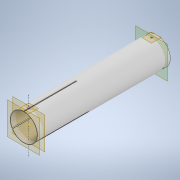
# Autodesk Inventor part: Segment_Engine
Saved by Autodesk Inventor 2020 (Build 240168000, 168)
## iProperties
Created: 2022-01-25
Part Number: Segment_Engine
Material: Generisch
Document SubType Name: Modeling
Designer: sp
Density: 1 g/cm^3
Appearance: Vorgabe
Author: sp
Autodesk Inventor part; units mm, degrees
ref_plane "YZ Plane" through (0, 0, 0) normal (1, 0, 0) x (0, 1, 0)
ref_plane "XZ Plane" through (0, 0, 0) normal (0, 1, 0) x (-1, 0, 0)
sketch "Skizze1" plane through (0, 0, 0) normal (0, 0, 1) x (1, 0, 0)
  circle A0 centre (0, 0) radius 31
  circle A1 centre (0, 0) radius 30
  dimension "d0" = 62
  dimension "d1" = 60
  constraints: 2 centre point, 2 coincident
  measures "d0" diameter of A0
  measures "d1" diameter of A1
extrude "Extrusion1" add sketch "Skizze1" along normal mid plane 300
ref_plane "Arbeitsebene1" through (0, 0, 138.75) normal (0, 0, 1) x (1, 0, 0)
sketch "Skizze2" plane through (0, 0, 138.75) normal (0, 0, 1) x (1, 0, 0)
  line L0 (0, 58.8638) -> (0, -62.7478) construction
  circle A0 centre (0, 0) radius 31 construction
  point P0 (0, 31)
  constraints: 2 end point, 1 point on line, 1 vertical, 1 vertical alignment, 1 other
ref_plane "Arbeitsebene2" through (0, 31, 138.75) normal (0, 1, 0) x (-1, 0, 0)
sketch "Skizze3" plane through (0, 31, 138.75) normal (0, 1, 0) x (-1, 0, 0)
  circle A0 centre (0, 0) radius 1.75
  line L0 (-43.4, 0) -> (43.4, 0) projected
  point P0 (0, -138.75)
  dimension "d5" = 3.5
  constraints: 1 centre point, 1 midpoint
  measures "d5" diameter of A0
extrude "Extrusion2" cut sketch "Skizze3" against normal blind 10
pattern_circular "Runde Anordnung1" count 3 over 360 about axis through (0, 0, -10) along (0, 0, 1) of "Extrusion2"
mirror "Spiegeln1" about plane through (0, 0, 0) normal (0, 0, 1) of "Extrusion2", "Runde Anordnung1"
ref_plane "Arbeitsebene5" through (0, 0, 151) normal (0, 0, 1) x (1, 0, 0)
sketch "Skizze4" plane through (0, 0, 151) normal (0, 0, 1) x (1, 0, 0)
  line L0 (-1, 29) -> (1, 29)
  line L1 (1, 29) -> (1, 33)
  line L2 (1, 33) -> (-1, 33)
  line L3 (-1, 33) -> (-1, 29)
  line L4 (0, 35.4216) -> (0, -14.4128) construction
  line L5 (-24.6147, -15.366) -> (-25.6147, -13.634)
  line L6 (-25.6147, -13.634) -> (-29.0788, -15.634)
  line L7 (-29.0788, -15.634) -> (-28.0788, -17.366)
  line L8 (-28.0788, -17.366) -> (-24.6147, -15.366)
  line L9 (25.6147, -13.634) -> (24.6147, -15.366)
  line L10 (24.6147, -15.366) -> (28.0788, -17.366)
  line L11 (28.0788, -17.366) -> (29.0788, -15.634)
  line L12 (29.0788, -15.634) -> (25.6147, -13.634)
  point P0 (0, 0)
  point P1 (-30.676, -17.7108)
  point P2 (30.676, -17.7108)
  dimension "d12" = 2
  dimension "d13" = 33
  dimension "d14" = 4
  dimension "d17" = 360
  constraints: 26 end point, 2 parallel, 1 horizontal, 1 perpendicular, 1 point on line, 1 vertical, 29 other
  measures "d12" distance of L0.start L0.end
  measures "d13" distance from line of point (0, 0) L2
  measures "d14" distance of L2.end L0.start
extrude "Extrusion3" cut sketch "Skizze4" against normal blind 120
ref_plane "Arbeitsebene3" through (0, 0, -138.75) normal (0, 0, 1) x (1, 0, 0)
ref_plane "Arbeitsebene4" through (0, 31, -138.75) normal (0, -1, 0) x (-1, 0, 0)
